led spacer_v4 (Autodesk Fusion 360 design; units mm, degrees)
Autodesk Fusion 360 part; units mm, degrees
sketch "Sketch1" plane through (0, 0, 0) normal (0, 1, 0) x (1, 0, 0)
  circle A0 centre (0, 0) radius 2.6289 construction
  circle A1 centre (0, 0) radius 2.9997 construction
  circle A2 centre (0, 0) radius 3.5077
  circle A3 centre (0, 0) radius 2.6924
  circle A4 centre (0, 0) radius 2.5006 construction
  dimension "d1" = 5.2578
  dimension "d2" = 5.9995
  dimension "d3" = 0.508
  dimension "d4" = 5.3848
  dimension "d5" = 5.0013
  constraint coincident A0.centre A1.centre
  constraint concentric A0 A1
  constraint concentric A1 A2
  constraint concentric A1 A3
  constraint concentric A2 A4
  measures "d1" diameter of A0
  measures "d2" diameter of A1
  measures "d3" distance of A1 A2
  measures "d4" diameter of A3
  measures "d5" diameter of A4
extrude "Extrude1" add sketch "Sketch1" along normal blind 1.27
equation "d1 = 0.1969 in + 0.0101 in"
equation "d4 = 0.1969 in + 0.0151 in"
equation "d6 = 0.2 in - 0.15 in"
